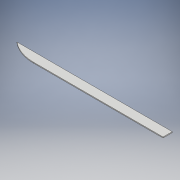
# Autodesk Inventor part: Part1
Saved by Autodesk Inventor 2018 (Build 220112000, 112)
## iProperties
Created: 2018-06-07
Part Number: Part1
Material: 一般
Document SubType Name: Modeling
Designer: ku_sk
Density: 1 g/cm^3
Appearance: 既定
Author: ku_sk
Autodesk Inventor part; units mm, degrees
ref_plane "YZ Plane" through (0, 0, 0) normal (1, 0, 0) x (0, 1, 0)
ref_plane "XZ Plane" through (0, 0, 0) normal (0, 1, 0) x (-1, 0, 0)
ref_plane "XY Plane" through (0, 0, 0) normal (0, 0, 1) x (1, 0, 0)
sketch "スケッチ1" plane through (0, 0, 0) normal (0, 0, 1) x (1, 0, 0)
  arc A0 (-240.8544, 35) -> (-160, 6) centre (-160, 133.2143) ccw projected
  line L0 (250, 6) -> (-160, 6) projected
  line L1 (250, 6) -> (250, 35) projected
  line L2 (250, 35) -> (-240.8544, 35) projected
  point P0 (0, 0)
extrude "押し出し1" add sketch "スケッチ1" along normal blind 3
